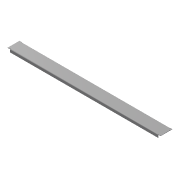
# Autodesk Inventor part: Деталь129
Saved by Autodesk Inventor 2017 (Build 210142000, 142)
## iProperties
Created: 2018-07-04
Part Number: Деталь129
Material: Сталь
Document SubType Name: Sheet Metal
Designer: Евтушенко
Mass: 6256.27 g
Surface Area: 5387.28 cm^2
Volume: 796.978 cm^3
Density: 7.85 g/cm^3
Sheet Metal Rule: ЧЗСК 1 мм
Appearance: Сталь
Author: Евтушенко
Autodesk Inventor part; units mm, degrees
note: some values were not read from the file. Chosen so that the rebuilt part matches the saved one: relief shape of "Пластина3"; relief shape of "Пластина4".
ref_plane "YZ Plane" through (0, 0, 0) normal (1, 0, 0) x (0, 1, 0)
ref_plane "XZ Plane" through (0, 0, 0) normal (0, 1, 0) x (-1, 0, 0)
ref_plane "XY Plane" through (0, 0, 0) normal (0, 0, 1) x (1, 0, 0)
sketch "Эскиз5" plane through (0, 0, 0) normal (0, 0, 1) x (1, 0, 0)
  line L0 (-258, -20) -> (258, -20)
  line L1 (258, -20) -> (258, 20)
  line L2 (258, 20) -> (-258, 20)
  line L3 (-258, 20) -> (-258, -20)
  line L4 (-258, -20) -> (258, 20) construction
  line L5 (258, -20) -> (-258, 20) construction
  point P0 (0, 0)
  dimension "d64" = 516
  dimension "d65" = 40
  measures "d64" distance of L2.end L1.end
  measures "d65" distance of L0.end L1.end
extrude "Пластина2" add sketch "Эскиз5" along normal blind 1
sketch "Эскиз6" plane through (258, 19, 1) normal (0, 1, 0) x (-1, 0, 0)
  line L0 (508, 0) -> (8, 0)
  line L1 (8, 0) -> (8, -10)
  line L2 (8, -10) -> (508, -10)
  line L3 (508, -10) -> (508, 0)
  constraints: 8 end point
edge flange "Фланец1" height 10 angle 90 thickness 1 bend radius 1.1 thickness toward (0, 1, 0) relief straight relief width 1 relief depth 0.5 edges at (0, 20, 0) wall of the first edge with corners at (-250, 19, 1) (250, 19, 1) (250, 19, -9) (-250, 19, -9)
bend "Сгиб1"
corner "УглСтык1"
sketch "Эскиз8" plane through (-258, -19, 1) normal (0, -1, 0) x (1, 0, 0)
  line L0 (508, 0) -> (8, 0)
  line L1 (8, 0) -> (8, -10)
  line L2 (8, -10) -> (508, -10)
  line L3 (508, -10) -> (508, 0)
  constraints: 8 end point
edge flange "Фланец2" height 10 angle 90 thickness 1 bend radius 1.1 thickness toward (0, -1, 0) relief straight relief width 1 relief depth 0.5 edges at (0, -20, 0) wall of the first edge with corners at (250, -19, 1) (-250, -19, 1) (-250, -19, -9) (250, -19, -9)
bend "Сгиб2"
corner "УглСтык2"
sketch "Эскиз7" plane through (0, 0, 1) normal (0, 0, 1) x (1, 0, 0)
  line L0 (-8.8388, -8.8388) -> (8.8388, 8.8388) construction
  line L1 (-7.0004, -10.6773) -> (10.6773, 7.0004)
  line L2 (7.0004, 10.6773) -> (-10.6773, -7.0004)
  arc A0 (-10.6773, -7.0004) -> (-7.0004, -10.6773) centre (-8.8388, -8.8388) ccw
  arc A1 (10.6773, 7.0004) -> (7.0004, 10.6773) centre (8.8388, 8.8388) ccw
  line L3 (0, 0) -> (25, 0) construction
  dimension "d77" = 45
  dimension "d78" = 25
  dimension "d79" = 2.6
  constraints: 10 end point, 4 point on circle, 4 tangent, 2 centre point, 1 equal length, 1 horizontal, 1 midpoint, 1 parallel
  measures "d77" angle of L3 L0
  measures "d78" distance of L0.start L0.end
  measures "d79" radius of A1
extrude "Вырез4" cut sketch "Эскиз7" against normal blind 1
pattern_linear "Прямоуг.массив1" count 16 spacing 15 along (1, 0, 0) count 16 spacing 15 along (-1, 0, 0) of "Вырез4"
equation "\"d80\" = Толщина"
equation "\"d67\" = Ширина_просечки"
equation "\"d68\" = Глубина_просечки"
equation "\"d69\" = Минимальный_остаток"
equation "\"d70\" = Радиус_гибки"
equation "\"d73\" = Радиус_гибки"
equation "\"d74\" = Размер_высечки"
equation "\"d75\" = Размер_зазора"
equation "\"d76\" = Радиус_Якоби"
equation "\"Ширина_просечки\" = Толщина"
equation "\"Глубина_просечки\" = 0.5 * Толщина"
equation "\"Размер_высечки\" = 4 * Толщина"
equation "\"Минимальный_остаток\" = 2 * Толщина"
equation "\"Радиус_перехода\" = Радиус_гибки"
equation "\"Радиус_Якоби\" = Радиус_гибки"
equation "\"Размер_зазора\" = Толщина"
equation "\"d2\" = Радиус_гибки"
equation "\"d66\" = Радиус_гибки"
equation "\"Толщина\" = 1"
equation "\"Радиус_гибки\" = 1.1"
